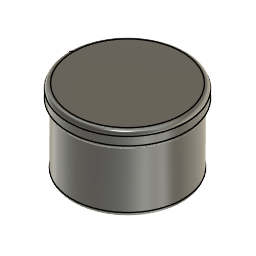
Threaded Container (Autodesk Fusion 360 design; units mm, degrees)
part number: 2026-08-12-00-50-46-556
Autodesk Fusion 360 part; units mm, degrees
sketch "Sketch1" plane through (0, 0, 0) normal (0, 0, 1) x (1, 0, 0)
  circle A0 centre (0, 0) radius 25
  dimension "d4" = 50
  constraint coincident A0.centre origin
  measures "d4" diameter of A0
extrude "Extrude1" add sketch "Sketch1" along normal blind 30 makes body 1
extrude "Extrude2" add 1 faces at (-6.7759, -1.242, 30) along direction (0, 0, 1) blind 3 separate body on bodies 1 makes body 2
move_face "OffsetFaces1" offset 1.4434 2 faces at (-24.9689, 1.2461, 31) (-6.7759, -1.242, 33) on bodies 2
extrude "Extrude3" cut 1 faces at (-6.7759, -1.242, 30) along direction (0, 0, 1) blind 3 on bodies 1 bodies 2
shell "Shell1" thickness 3 removed faces 1 at (-6.7759, -1.242, 30) on bodies 1
thread "Thread1" "ISO Metric profile 50.0 M50x3 M50x3 6g" major diameter 49.7645 minor diameter 46.3239 pitch 3 angle 60 modelled right hand crest width 0.422 on face at (24.8758, -2.4892, 20) from (0, 0, 27) to (0, 0, 30) crest through (24.8822, 0, -0.75) on bodies 1
thread "Thread2" "ISO Metric profile 50.0 M50x3 M50x3 6H" major diameter 50.3564 minor diameter 47.0024 pitch 3 angle 60 modelled right hand crest width 0.8135 on face at (24.9689, -1.2461, 32) crest through (23.5012, 0, 30.75) on bodies 2
move_body "Move1" bodies 2 to x (1, 0, 0) y (0, 1, 0) z (0, 0, 1) at (0, 0, -3)
ref_plane "WorkPlane2" through (0, 0, 27) normal (0, 0, -1) x (-1, 0, 0)
split "Split1" by plane through (0, 0, 27) normal (0, 0, -1) bodies 1 makes body 3 at (0, 24.8822, 9)
scale "Scale2" factors (1, 1, 1.732051) about (-17.6858, -15.4763, 27) bodies 2 1
move_body "Move4" bodies 2 to x (1, 0, 0) y (0, 1, 0) z (0, 0, 1) at (0, 0, 0)
combine "Combine1" operation add target body 1 tool bodies 3
fillet "Fillet2" radius 2 curvature continuous 3 edges at (-23.1984, -8.9978, 0) (-24.6539, -9.5623, 34.6962) (-24.6539, -9.5623, 27) on bodies 1 2
equation "ThreadHeight = 3 mm"
equation "containerHeight = 30 mm"
equation "containerWidth = 50 mm"
equation "d4 = containerWidth"
equation "d5 = containerHeight"
equation "d7 = ThreadHeight"
equation "d9 = LidThickness * ( sqrt(1 / 3) )"
equation "d10 = ThreadHeight"
equation "d14 = ThreadHeight"
equation "d19 = -ThreadHeight"
equation "filletRadius = 2 mm"
equation "LidThickness = 2.5 mm"
equation "d36 = sqrt(3)"
